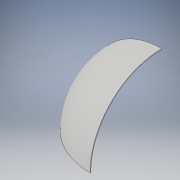
# Autodesk Inventor part: shell
Saved by Autodesk Inventor 2019 (Build 230136000, 136)
## iProperties
Created: 2019-02-10
Part Number: shell
Material: Generic
Document SubType Name: Modeling
Designer: mashimaro
Density: 1 g/cm^3
Appearance: Default
Author: mashimaro
Autodesk Inventor part; units mm, degrees
ref_plane "YZ Plane" through (0, 0, 0) normal (1, 0, 0) x (0, 1, 0)
ref_plane "XZ Plane" through (0, 0, 0) normal (0, 1, 0) x (-1, 0, 0)
ref_plane "XY Plane" through (0, 0, 0) normal (0, 0, 1) x (1, 0, 0)
sketch "Sketch1" plane through (0, 0, 0) normal (0, 1, 0) x (-1, 0, 0)
  arc A0 (172, 0) -> (0, 172) centre (0, 0) ccw
  line L0 (0, 172) -> (0, 0)
  line L1 (172, 0) -> (0, 0)
  constraints: 4 end point, 2 point on circle, 1 centre point, 1 horizontal, 1 vertical
revolve "Revolution1" add sketch "Sketch1" angle 90 about axis through (0, 0, 172) along (0, 0, -1)
sketch "Sketch2" plane through (-172, 0, 0) normal (0, -1, 0) x (1, 0, 0)
  arc A0 (172, 170) -> (2, 0) centre (172, 0) ccw
  line L0 (172, 0) -> (172, 172) projected
  line L1 (172, 0) -> (2, 0)
  line L2 (172, 0) -> (172, 170)
  constraints: 4 end point, 2 point on circle, 1 centre point, 1 coincident, 1 perpendicular, 1 point on line
revolve "Revolution2" cut sketch "Sketch2" angle 90 about axis through (0, 0, 0) along (0, 0, -1)
body "Solid1"
